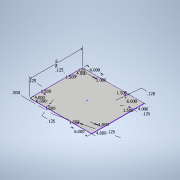
# Autodesk Inventor part: seatfloorfit
Saved by Autodesk Inventor 2021 (Build 250183000, 183)
## iProperties
Created: 2020-10-26
Part Number: seatfloorfit
Material: Generic
Document SubType Name: Modeling
Designer: mackeycj
Density: 1 g/cm^3
Appearance: Default
Author: mackeycj
Autodesk Inventor part; units mm, degrees
ref_plane "YZ Plane" through (0, 0, 0) normal (1, 0, 0) x (0, 1, 0)
ref_plane "XZ Plane" through (0, 0, 0) normal (0, 1, 0) x (-1, 0, 0)
ref_plane "XY Plane" through (0, 0, 0) normal (0, 0, 1) x (1, 0, 0)
sketch "Sketch1" plane through (0, 0, 0) normal (0, 1, 0) x (-1, 0, 0)
  line L0 (-292.1, -248.92) -> (292.1, -248.92)
  line L1 (292.1, -248.92) -> (292.1, 248.92)
  line L2 (292.1, 248.92) -> (-292.1, 248.92)
  line L3 (-292.1, 248.92) -> (-292.1, -248.92)
  line L4 (-292.1, -248.92) -> (292.1, 248.92) construction
  line L5 (292.1, -248.92) -> (-292.1, 248.92) construction
  point P0 (0, 0)
  dimension "d0" = 584.2
  dimension "d1" = 497.84
  constraints: 12 end point, 2 midpoint, 2 parallel, 1 horizontal, 1 perpendicular
  measures "d0" distance of L2.end L1.end
  measures "d1" distance of L1.end L0.end
extrude "Extrusion1" add sketch "Sketch1" along normal blind 1.524
sketch "Sketch3" plane through (0, 0, 0) normal (1, 0, 0) x (0, 1, 0)
  point P0 (0, 0)
sketch "Sketch4" plane through (0, 0, 0) normal (0, 1, 0) x (-1, 0, 0)
  line L0 (292.1, 248.92) -> (-292.1, 248.92) projected
  line L1 (292.1, 248.92) -> (292.1, 147.32)
  line L2 (292.1, -248.92) -> (292.1, 248.92) projected
  line L3 (292.1, 147.32) -> (254, 147.32)
  circle A0 centre (254, 147.32) radius 6.35
  line L4 (292.1, -248.92) -> (292.1, -147.32)
  line L5 (292.1, -147.32) -> (254, -147.32)
  circle A1 centre (254, -147.32) radius 6.35
  line L6 (-292.1, -248.92) -> (292.1, -248.92) projected
  line L7 (292.1, -248.92) -> (139.7, -248.92)
  line L8 (139.7, -248.92) -> (101.6, -248.92)
  circle A2 centre (139.7, -223.52) radius 6.35
  line L9 (-292.1, 248.92) -> (-292.1, -248.92) projected
  line L10 (-292.1, -248.92) -> (-139.7, -248.92)
  line L11 (-139.7, -248.92) -> (-139.7, -210.82)
  circle A3 centre (-139.7, -223.52) radius 6.35
  line L12 (-292.1, -248.92) -> (-292.1, -147.32)
  line L13 (-292.1, -147.32) -> (-254, -147.32)
  line L14 (-292.1, 248.92) -> (-292.1, 147.32)
  line L15 (-292.1, 147.32) -> (-254, 147.32)
  line L16 (-292.1, 248.92) -> (-139.7, 248.92)
  line L17 (-139.7, 248.92) -> (-139.7, 223.52)
  circle A4 centre (-139.7, 223.52) radius 6.35
  line L18 (292.1, 248.92) -> (139.7, 248.92)
  line L19 (139.7, 248.92) -> (139.7, 223.52)
  circle A5 centre (139.7, 223.52) radius 6.35
  circle A6 centre (-254, 147.32) radius 6.35
  circle A7 centre (-254, -147.32) radius 6.35
  line L20 (139.7, -248.92) -> (139.7, -223.52)
  point P0 (0, 0)
  dimension "d10" = 101.6
  dimension "d11" = 38.1
  dimension "d12" = 12.7
  dimension "d13" = 101.6
  dimension "d14" = 38.1
  dimension "d15" = 12.7
  dimension "d16" = 152.4
  dimension "d18" = 12.7
  dimension "d19" = 152.4
  dimension "d20" = 38.1
  dimension "d21" = 12.7
  dimension "d22" = 101.6
  dimension "d23" = 38.1
  dimension "d24" = 101.6
  dimension "d25" = 38.1
  dimension "d26" = 152.4
  dimension "d27" = 25.4
  dimension "d28" = 12.7
  dimension "d29" = 152.4
  dimension "d30" = 25.4
  dimension "d31" = 12.7
  dimension "d32" = 12.7
  dimension "d33" = 12.7
  dimension "d39" = 25.4
  constraints: 34 end point, 9 point on line, 8 centre point, 6 coincident, 6 perpendicular, 1 horizontal, 1 vertical
  measures "d10" distance of L0.start L1.end
  measures "d11" distance of L1.end L3.end
  measures "d12" diameter of A0
  measures "d13" distance of L2.start L4.end
  measures "d14" distance of L4.end L5.end
  measures "d15" diameter of A1
  measures "d16" distance of L2.start L7.end
  measures "d18" diameter of A2
  measures "d19" distance of L6.start L10.end
  measures "d20" distance of L10.end L11.end
  measures "d21" diameter of A3
  measures "d22" distance of L6.start L12.end
  measures "d23" distance of L12.end L13.end
  measures "d24" distance of L0.end L14.end
  measures "d25" distance of L14.end L15.end
  measures "d26" distance of L0.end L16.end
  measures "d27" distance of L16.end L17.end
  measures "d28" diameter of A4
  measures "d29" distance of L0.start L18.end
  measures "d30" distance of L18.end L19.end
  measures "d31" diameter of A5
  measures "d32" diameter of A6
  measures "d33" diameter of A7
  measures "d39" distance of L7.end L20.end
extrude "Extrusion3" cut sketch "Sketch4" along normal blind 25.4 contours A5 | A4 | A6 | A7 | A3 L11 | L11 A3 | A2 | A1 | A0
sketch "Sketch5" plane through (0, 0, 0) normal (0, 1, 0) x (-1, 0, 0)
  line L0 (292.1, 248.92) -> (-292.1, 248.92)
  line L1 (292.1, 248.92) -> (292.1, 147.32)
  line L2 (292.1, -248.92) -> (292.1, 248.92)
  line L3 (292.1, 147.32) -> (254, 147.32)
  circle A0 centre (254, 147.32) radius 1.5875
  line L4 (292.1, -248.92) -> (292.1, -147.32)
  line L5 (292.1, -147.32) -> (254, -147.32)
  circle A1 centre (254, -147.32) radius 1.5875
  line L6 (-292.1, -248.92) -> (292.1, -248.92)
  line L7 (292.1, -248.92) -> (139.7, -248.92)
  line L8 (139.7, -248.92) -> (101.6, -248.92)
  circle A2 centre (139.7, -223.52) radius 1.5875
  line L9 (-292.1, 248.92) -> (-292.1, -248.92)
  line L10 (-292.1, -248.92) -> (-139.7, -248.92)
  line L11 (-139.7, -248.92) -> (-139.7, -210.82)
  circle A3 centre (-139.7, -223.52) radius 1.6256
  line L12 (-292.1, -248.92) -> (-292.1, -147.32)
  line L13 (-292.1, -147.32) -> (-254, -147.32)
  line L14 (-292.1, 248.92) -> (-292.1, 147.32)
  line L15 (-292.1, 147.32) -> (-254, 147.32)
  line L16 (-292.1, 248.92) -> (-139.7, 248.92)
  line L17 (-139.7, 248.92) -> (-139.7, 223.52)
  circle A4 centre (-139.7, 223.52) radius 6.35
  line L18 (292.1, 248.92) -> (139.7, 248.92)
  line L19 (139.7, 248.92) -> (139.7, 223.52)
  circle A5 centre (139.7, 223.52) radius 1.5875
  circle A6 centre (-254, 147.32) radius 1.5875
  circle A7 centre (-254, -147.32) radius 1.5875
  line L20 (139.7, -248.92) -> (139.7, -223.52)
  point P0 (0, 0)
  point P1 (0, 0)
  dimension "d42" = 101.6
  dimension "d43" = 38.1
  dimension "d44" = 3.175
  dimension "d45" = 101.6
  dimension "d46" = 38.1
  dimension "d47" = 3.175
  dimension "d48" = 152.4
  dimension "d49" = 3.175
  dimension "d50" = 152.4
  dimension "d51" = 38.1
  dimension "d52" = 3.2512
  dimension "d53" = 101.6
  dimension "d54" = 38.1
  dimension "d55" = 101.6
  dimension "d56" = 38.1
  dimension "d57" = 152.4
  dimension "d58" = 25.4
  dimension "d59" = 12.7
  dimension "d60" = 152.4
  dimension "d61" = 25.4
  dimension "d62" = 3.175
  dimension "d63" = 3.175
  dimension "d64" = 3.175
  dimension "d65" = 25.4
  constraints: 42 end point, 9 point on line, 8 centre point, 6 coincident, 6 perpendicular, 1 horizontal, 1 vertical
  measures "d42" distance of L0.start L1.end
  measures "d43" distance of L1.end L3.end
  measures "d44" diameter of A0
  measures "d45" distance of L2.start L4.end
  measures "d46" distance of L4.end L5.end
  measures "d47" diameter of A1
  measures "d48" distance of L2.start L7.end
  measures "d49" diameter of A2
  measures "d50" distance of L6.start L10.end
  measures "d51" distance of L10.end L11.end
  measures "d52" diameter of A3
  measures "d53" distance of L6.start L12.end
  measures "d54" distance of L12.end L13.end
  measures "d55" distance of L0.end L14.end
  measures "d56" distance of L14.end L15.end
  measures "d57" distance of L0.end L16.end
  measures "d58" distance of L16.end L17.end
  measures "d59" diameter of A4
  measures "d60" distance of L0.start L18.end
  measures "d61" distance of L18.end L19.end
  measures "d62" diameter of A5
  measures "d63" diameter of A6
  measures "d64" diameter of A7
  measures "d65" distance of L7.end L20.end
body "Solid1"
